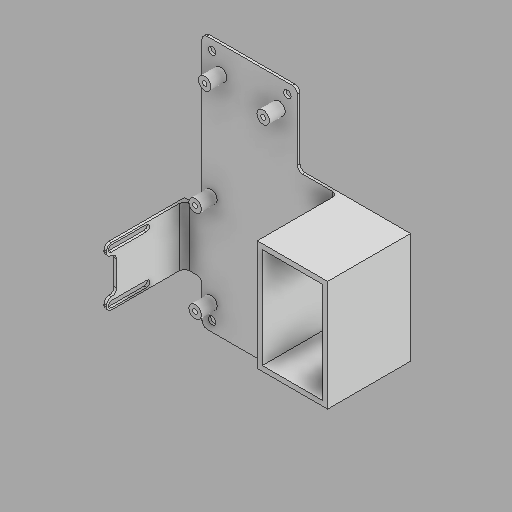
# Autodesk Inventor part: RC_CAR_CONTROLLER_PLATE
Saved by Autodesk Inventor 2025.2 (Build 292293000, 293)
## iProperties
Created: 2025-10-28
Part Number: RC_CAR_CONTROLLER_PLATE
Material: Generic
Document SubType Name: Modeling
Designer: Ben
Density: 1 g/cm^3
Appearance: Default
Author: Ben
Autodesk Inventor part; units mm, degrees
ref_plane "YZ Plane" through (0, 0, 0) normal (1, 0, 0) x (0, 1, 0)
ref_plane "XZ Plane" through (0, 0, 0) normal (0, 1, 0) x (-1, 0, 0)
ref_plane "XY Plane" through (0, 0, 0) normal (0, 0, 1) x (1, 0, 0)
sketch "Sketch1" plane through (0, 0, 0) normal (0, 0, 1) x (1, 0, 0)
  line L0 (-30.1625, -80.1688) -> (30.1625, -80.1688)
  line L1 (30.1625, -80.1688) -> (30.1625, 80.1688)
  line L2 (30.1625, 80.1688) -> (-30.1625, 80.1688)
  line L3 (-30.1625, 80.1688) -> (-30.1625, -80.1688)
  line L4 (-30.1625, -80.1688) -> (30.1625, 80.1688) construction
  line L5 (30.1625, -80.1688) -> (-30.1625, 80.1688) construction
  point P0 (0, 0)
  dimension "d0" = 160.3375
  dimension "d1" = 60.325
  constraints: 12 end point, 2 midpoint, 2 parallel, 1 horizontal, 1 perpendicular
  measures "d0" distance of L0.end L1.end
  measures "d1" distance of L1.end L2.end
extrude "Extrusion1" add sketch "Sketch1" along normal blind 1.5875
sketch "Sketch3" plane through (0, 0, 1.5875) normal (0, 0, 1) x (1, 0, 0)
  circle A0 centre (-24.5, -64.2938) radius 3.9688
  circle A1 centre (24.5, -64.2938) radius 3.9688
  line L0 (0, -112.2363) -> (0, 112.2363) projected
  line L1 (-42.2275, 0) -> (42.2275, 0) projected
  circle A2 centre (-24.5, -6.2937) radius 3.9688
  circle A3 centre (24.5, -6.2937) radius 3.9688
  circle A4 centre (-18.5, 63.5563) radius 3.9688
  circle A5 centre (18.5, 63.5563) radius 3.9688
  line L2 (-30.1625, -80.1688) -> (30.1625, -80.1688) projected
  point P0 (0, 0)
  dimension "d4" = 49
  dimension "d5" = 58
  dimension "d6" = 37
  dimension "d7" = 15.875
  dimension "d8" = 7.9375
  dimension "d9" = 69.85
  constraints: 6 centre point, 2 equal radius, 2 vertical alignment, 1 horizontal alignment, 3 other
  measures "d4" distance of A1.centre A0.centre
  measures "d5" distance of A1.centre A3.centre
  measures "d6" distance of A5.centre A4.centre
  measures "d7" distance from line of L2 A1.centre
  measures "d8" diameter of A3
  measures "d9" vertical distance of A3.centre A5.centre
extrude "Extrusion2" add sketch "Sketch3" along normal blind 10
sketch "Sketch4" plane through (0, 0, 1.5875) normal (0, 0, 1) x (1, 0, 0)
  line L0 (0, -112.2363) -> (0, 112.2363) projected
  line L1 (-42.2275, 0) -> (42.2275, 0) projected
  line L2 (-30.1625, 80.1688) -> (-30.1625, -80.1688) projected
  point P0 (0, 0)
  point P1 (-23.8125, 73.8187)
  point P2 (-23.8125, -73.8187)
  point P3 (23.8125, -73.8187)
  point P4 (23.8125, 73.8187)
  dimension "d12" = 147.6375
  dimension "d13" = 6.35
  constraints: 3 symmetric about line, 2 vertical alignment
  measures "d12" distance of point (-23.812, 73.819) point (-23.812, -73.819)
  measures "d13" distance from line of L2 point (-23.812, -73.819)
hole "Hole1" at (-23.8125, 73.8187, 1.5875) at (-23.8125, -73.8187, 1.5875) at (23.8125, -73.8187, 1.5875) at (23.8125, 73.8187, 1.5875) direction (0, 0, -1) diameter 4.7625 end through all
sketch "Sketch5" plane through (0, 0, 0) normal (0, 0, -1) x (-1, 0, 0)
  circle A0 centre (24.5, -64.2938) radius 3.9687 projected
  circle A1 centre (24.5, -6.2937) radius 3.9687 projected
  line L0 (24.5, -64.2938) -> (24.5, -6.2937) construction
  line L1 (30.1625, 80.1688) -> (30.1625, -80.1688) projected
  line L2 (42.8625, -16.8687) -> (30.1625, -16.8687)
  line L3 (30.1625, -16.8687) -> (30.1625, -53.7188)
  line L4 (30.1625, -53.7188) -> (42.8625, -53.7188)
  line L5 (42.8625, -53.7188) -> (42.8625, -16.8687)
  line L6 (42.8625, -16.8687) -> (30.1625, -53.7188) construction
  line L7 (30.1625, -16.8687) -> (42.8625, -53.7188) construction
  point P0 (0, 0)
  point P1 (36.5125, -35.2938)
  point P2 (24.5, -35.2938)
  dimension "d21" = 12.7
  dimension "d22" = 36.85
  constraints: 14 end point, 3 midpoint, 2 parallel, 1 horizontal, 1 horizontal alignment, 1 perpendicular, 1 point on line, 1 vertical
  measures "d21" distance between parallel lines of L1 L5
  measures "d22" distance between parallel lines of L2 L4
extrude "Extrusion3" add sketch "Sketch5" against normal blind 50.8 contours L2 L5 L4 L1
sketch "Sketch6" plane through (-42.8625, -53.7188, 0) normal (-1, 0, 0) x (0, 0, 1)
  line L0 (47.625, 33.675) -> (25.4, 33.675) construction
  line L1 (47.625, 35.675) -> (25.4, 35.675)
  line L2 (25.4, 31.675) -> (47.625, 31.675)
  arc A0 (47.625, 31.675) -> (47.625, 35.675) centre (47.625, 33.675) ccw
  arc A1 (25.4, 35.675) -> (25.4, 31.675) centre (25.4, 33.675) ccw
  line L3 (47.625, 3.175) -> (25.4, 3.175) construction
  line L4 (47.625, 5.175) -> (25.4, 5.175)
  line L5 (25.4, 1.175) -> (47.625, 1.175)
  arc A2 (47.625, 1.175) -> (47.625, 5.175) centre (47.625, 3.175) ccw
  arc A3 (25.4, 5.175) -> (25.4, 1.175) centre (25.4, 3.175) ccw
  line L6 (50.8, 0) -> (50.8, 36.85) construction
  line L7 (50.8, 18.425) -> (0, 18.425) construction
  line L8 (0, -26.45) -> (0, 133.8875) construction
  line L9 (44.45, 29.675) -> (50.8, 29.675)
  line L10 (50.8, 29.675) -> (50.8, 7.175)
  line L11 (50.8, 7.175) -> (44.45, 7.175)
  line L12 (44.45, 7.175) -> (44.45, 29.675)
  line L13 (44.45, 29.675) -> (50.8, 7.175) construction
  line L14 (50.8, 29.675) -> (44.45, 7.175) construction
  point P0 (0, 53.7188)
  point P1 (36.5125, 33.675)
  point P2 (36.5125, 3.175)
  point P3 (47.625, 18.425)
  dimension "d25" = 30.5
  dimension "d26" = 4
  dimension "d27" = 22.225
  dimension "d28" = 3.175
  dimension "d29" = 4
  dimension "d30" = 6.35
  constraints: 30 end point, 8 point on circle, 8 tangent, 5 midpoint, 5 parallel, 4 centre point, 3 horizontal, 3 point on line, 2 vertical alignment, 1 equal radius, 1 perpendicular, 1 other
  measures "d25" distance between parallel lines of L3 L0
  measures "d26" distance between parallel lines of L1 L2
  measures "d27" distance of L0.end L0.start
  measures "d28" distance from line of L6 L0.start
  measures "d29" distance between parallel lines of L0 L9
  measures "d30" distance of L10.end L11.end
extrude "Extrusion4" cut sketch "Sketch6" along normal through all both and the other way through all
sketch "Sketch7" plane through (0, 0, 0) normal (0, 0, -1) x (-1, 0, 0)
  line L0 (71.4375, 0) -> (-128.5875, 0) projected
  line L1 (0, -112.2363) -> (0, 112.2363) projected
  line L2 (-30.1625, -80.1688) -> (-30.1625, 80.1688) projected
  line L3 (-100.0125, -34.925) -> (-30.1625, -34.925)
  line L4 (-30.1625, -34.925) -> (-30.1625, 34.925)
  line L5 (-30.1625, 34.925) -> (-100.0125, 34.925)
  line L6 (-100.0125, 34.925) -> (-100.0125, -34.925)
  line L7 (-100.0125, -34.925) -> (-30.1625, 34.925) construction
  line L8 (-30.1625, -34.925) -> (-100.0125, 34.925) construction
  point P0 (0, 0)
  point P1 (-65.0875, 0)
  dimension "d33" = 69.85
  dimension "d34" = 69.85
  constraints: 12 end point, 2 midpoint, 2 parallel, 2 point on line, 1 horizontal, 1 perpendicular
  measures "d33" distance of L4.end L5.end
  measures "d34" distance of L5.end L3.start
extrude "Extrusion5" add sketch "Sketch7" against normal up to surface (1.5875 mm away)
sketch "Sketch8" plane through (0, 0, 1.5875) normal (0, 0, 1) x (1, 0, 0)
  line L0 (100.0125, -34.925) -> (30.1625, -34.925) projected
  line L1 (30.1625, 34.925) -> (100.0125, 34.925) projected
  line L2 (100.0125, -34.925) -> (55.5625, -34.925)
  line L3 (55.5625, -34.925) -> (55.5625, 34.925)
  line L4 (55.5625, 34.925) -> (100.0125, 34.925)
  line L5 (100.0125, 34.925) -> (100.0125, -34.925)
  point P0 (0, 0)
  dimension "d37" = 44.45
  constraints: 8 end point, 2 parallel, 1 horizontal, 1 perpendicular, 1 point on line
  measures "d37" distance between parallel lines of L5 L3
extrude "Extrusion6" add sketch "Sketch8" along normal blind 50.8
sketch "Sketch9" plane through (0, 0, 52.3875) normal (0, 0, 1) x (1, 0, 0)
  line L0 (100.0125, 34.925) -> (55.5625, 34.925) projected
  line L1 (55.5625, 34.925) -> (55.5625, -34.925) projected
  line L2 (55.5625, -34.925) -> (100.0125, -34.925) projected
  line L3 (100.0125, -34.925) -> (100.0125, 34.925) projected
  line L4 (96.8375, 31.75) -> (58.7375, 31.75)
  line L5 (58.7375, 31.75) -> (58.7375, -31.75)
  line L6 (58.7375, -31.75) -> (96.8375, -31.75)
  line L7 (96.8375, -31.75) -> (96.8375, 31.75)
  line L8 (96.8375, 31.75) -> (58.7375, -31.75) construction
  line L9 (58.7375, 31.75) -> (96.8375, -31.75) construction
  line L10 (-71.4375, 0) -> (128.5875, 0) projected
  line L11 (100.0125, -34.925) -> (30.1625, -34.925) construction
  line L12 (77.7875, -34.925) -> (77.7875, 34.925) construction
  point P0 (0, 0)
  point P1 (77.7875, 0)
  dimension "d40" = 3.175
  dimension "d41" = 3.175
  constraints: 14 end point, 3 midpoint, 2 parallel, 1 horizontal, 1 perpendicular, 1 point on line, 2 other
  measures "d40" distance between parallel lines of L2 L6
  measures "d41" distance between parallel lines of L3 L7
extrude "Extrusion7" cut sketch "Sketch9" against normal up to surface (50.8 mm away) contours L10 L5 L4 L7 | L7 L6 L5 L10
sketch "Sketch10" plane through (18.5, 63.5563, 11.5875) normal (0, 0, 1) x (1, 0, 0)
  circle A0 centre (6, -69.85) radius 3.9687 projected
  circle A1 centre (-43, -69.85) radius 3.9687 projected
  circle A2 centre (-37, 0) radius 3.9687 projected
  circle A3 centre (6, -127.85) radius 3.9687 projected
  circle A4 centre (-43, -127.85) radius 3.9687 projected
  circle A5 centre (0, 0) radius 3.9687 projected
  point P0 (-18.5, -63.5563)
  constraints: 6 coincident
hole "Hole2" at (18.5, 63.5563, 11.5875) at (-18.5, 63.5563, 11.5875) at (24.5, -6.2938, 11.5875) at (-24.5, -6.2938, 11.5875) at (24.5, -64.2937, 11.5875) at (-24.5, -64.2937, 11.5875) direction (0, 0, -1) diameter 3 depth 10 tip angle 118
sketch "Sketch11" plane through (-30.1625, -53.7188, 1.5875) normal (1, 0, 0) x (0, 0, -1)
  line L0 (0, 0) -> (-49.2125, 0) projected
  line L1 (-49.2125, 29.675) -> (-49.2125, 36.85) projected
  line L2 (0, 0) -> (-49.2125, 0)
  line L3 (-49.2125, 0) -> (-49.2125, 36.85)
  line L4 (-49.2125, 36.85) -> (0, 36.85)
  line L5 (0, 36.85) -> (0, 0)
  point P0 (1.5875, 53.7187)
  constraints: 8 end point, 2 parallel, 1 horizontal, 1 perpendicular
extrude "Extrusion8" cut sketch "Sketch11" against normal blind 11.1125
fillet "Fillet2" radius 3.175 16 edges at (-41.275, -35.2938, 1.5875) (-30.1625, -16.8687, 0.7937) (-30.1625, 80.1688, 0.7937) (30.1625, 80.1688, 0.7937) (30.1625, 34.925, 0.7937) (55.5625, 0, 1.5875) (30.1625, -34.925, 0.7937) (30.1625, -80.1688, 0.7937) (-30.1625, -80.1688, 0.7937) (-30.1625, -53.7188, 0.7937) (-42.0687, -53.7188, 50.8) (-42.0687, -46.5437, 50.8) (-42.0687, -46.5438, 44.45) (-42.0687, -24.0437, 44.45) (-42.0687, -24.0437, 50.8) (-42.0687, -16.8687, 50.8)
body "Solid1"
